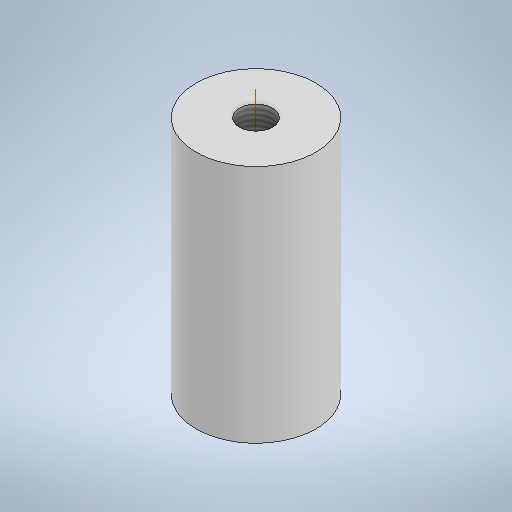
# Autodesk Inventor part: mocowanie_pod_hak
Saved by Autodesk Inventor 2025.2 (Build 292293000, 293)
## iProperties
Created: 2025-04-28
Part Number: mocowanie_pod_hak
Material: Ogólny
Document SubType Name: Modeling
Designer: marci
Density: 1 g/cm^3
Appearance: Domyślna
Author: marci
Autodesk Inventor part; units mm, degrees
ref_plane "YZ Plane" through (0, 0, 0) normal (1, 0, 0) x (0, 1, 0)
ref_plane "XZ Plane" through (0, 0, 0) normal (0, 1, 0) x (-1, 0, 0)
ref_plane "XY Plane" through (0, 0, 0) normal (0, 0, 1) x (1, 0, 0)
sketch "Szkic1" plane through (0, 0, 0) normal (0, 1, 0) x (-1, 0, 0)
  circle A0 centre (0, 0) radius 25
  constraints: 1 centre point, 1 coincident
extrude "Wyciągnięcie proste1" add sketch "Szkic1" along normal blind 100
sketch "Szkic2" plane through (0, 0, 0) normal (0, -1, 0) x (1, 0, 0)
  circle A0 centre (0, 0) radius 25 projected
  constraints: 1 coincident
hole "Otwór1" at (0, 0, 0) direction (0, 1, 0) diameter 13.835 depth 41.3 tip angle 118 thread size "M16x2" class "6H" standard "ISO Metric profile"
sketch "Szkic3" plane through (0, 100, 0) normal (0, 1, 0) x (1, 0, 0)
  line L0 (0, 0) -> (-13.3904, -21.1115)
  circle A0 centre (0, 0) radius 25 projected
  constraints: 2 end point, 2 other
hole "Otwór2" at (0, 100, 0) direction (0, -1, 0) diameter 13.835 depth 41.3 tip angle 118 thread size "M16x2" class "6H" standard "ISO Metric profile"
